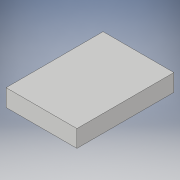
# Autodesk Inventor part: outer_heatsink
Saved by Autodesk Inventor 2017 (Build 210142000, 142)
## iProperties
Created: 2018-03-08
Part Number: outer_heatsink
Material: Generic
Document SubType Name: Modeling
Designer: Zara
Density: 1 g/cm^3
Appearance: Default
Author: Zara
Autodesk Inventor part; units mm, degrees
ref_plane "YZ Plane" through (0, 0, 0) normal (1, 0, 0) x (0, 1, 0)
ref_plane "XZ Plane" through (0, 0, 0) normal (0, 1, 0) x (-1, 0, 0)
ref_plane "XY Plane" through (0, 0, 0) normal (0, 0, 1) x (1, 0, 0)
sketch "Sketch1" plane through (0, 0, 0) normal (0, 1, 0) x (-1, 0, 0)
  line L0 (53.7845, 53.7845) -> (-53.7845, 53.7845)
  line L1 (-53.7845, 53.7845) -> (-53.7845, -93.5355)
  line L2 (-53.7845, -93.5355) -> (53.7845, -93.5355)
  line L3 (53.7845, -93.5355) -> (53.7845, 53.7845)
  point P0 (0, 0)
  dimension "d0" = 107.569
  dimension "d1" = 147.32
  constraints: 8 end point, 2 parallel, 1 horizontal, 1 perpendicular
  measures "d0" distance of L0.start L0.end
  measures "d1" distance of L2.end L0.start
extrude "Extrusion1" add sketch "Sketch1" along normal blind 26.035
body "Solid1"
